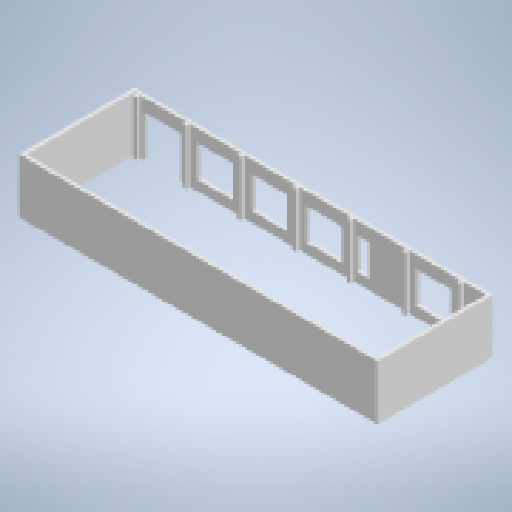
# Autodesk Inventor part: Part1
Saved by Autodesk Inventor 2024.2 (Build 282272000, 272)
## iProperties
Created: 2024-04-05
Part Number: Part1
Material: Generic
Document SubType Name: Modeling
Designer: admin
Density: 1 g/cm^3
Appearance: Default
Author: admin
Autodesk Inventor part; units mm, degrees
ref_plane "YZ Plane" through (0, 0, 0) normal (1, 0, 0) x (0, 1, 0)
ref_plane "XZ Plane" through (0, 0, 0) normal (0, 1, 0) x (-1, 0, 0)
ref_plane "XY Plane" through (0, 0, 0) normal (0, 0, 1) x (1, 0, 0)
sketch "Sketch1" plane through (0, 0, 0) normal (0, 1, 0) x (-1, 0, 0)
  line L0 (19320, -5950) -> (-19320, -5950)
  line L1 (-19320, -5950) -> (-19320, 5950)
  line L2 (-19320, 5950) -> (19320, 5950)
  line L3 (19320, 5950) -> (19320, -5950)
  line L4 (19320, -5950) -> (-19320, 5950) construction
  line L5 (-19320, -5950) -> (19320, 5950) construction
  line L6 (-19720, -6350) -> (19720, -6350)
  line L7 (19720, -6350) -> (19720, 6350)
  line L8 (19720, 6350) -> (-19720, 6350)
  line L9 (-19720, 6350) -> (-19720, -6350)
  line L10 (-16470, -5950) -> (-16870, -5950)
  line L11 (-16870, -5950) -> (-16870, -5550)
  line L12 (-16870, -5550) -> (-16470, -5550)
  line L13 (-16470, -5550) -> (-16470, -5950)
  line L14 (-16470, -5950) -> (-16870, -5550) construction
  line L15 (-16870, -5950) -> (-16470, -5550) construction
  line L16 (-16470, 5850) -> (-16870, 5850)
  line L17 (-16870, 5850) -> (-16870, 5950)
  line L18 (-16870, 5950) -> (-16470, 5950)
  line L19 (-16470, 5950) -> (-16470, 5850)
  line L20 (-16470, 5850) -> (-16870, 5950) construction
  line L21 (-16870, 5850) -> (-16470, 5950) construction
  line L22 (-10499, -5950) -> (-10899, -5950)
  line L23 (-10899, -5950) -> (-10899, -5550)
  line L24 (-10899, -5550) -> (-10499, -5550)
  line L25 (-10499, -5550) -> (-10499, -5950)
  line L26 (-10499, -5950) -> (-10899, -5550) construction
  line L27 (-10899, -5950) -> (-10499, -5550) construction
  line L28 (-4427, -5950) -> (-4827, -5950)
  line L29 (-4827, -5950) -> (-4827, -5550)
  line L30 (-4827, -5550) -> (-4427, -5550)
  line L31 (-4427, -5550) -> (-4427, -5950)
  line L32 (-4427, -5950) -> (-4827, -5550) construction
  line L33 (-4827, -5950) -> (-4427, -5550) construction
  line L34 (1573, -5950) -> (1173, -5950)
  line L35 (1173, -5950) -> (1173, -5550)
  line L36 (1173, -5550) -> (1573, -5550)
  line L37 (1573, -5550) -> (1573, -5950)
  line L38 (1573, -5950) -> (1173, -5550) construction
  line L39 (1173, -5950) -> (1573, -5550) construction
  line L40 (7598, -5950) -> (7198, -5950)
  line L41 (7198, -5950) -> (7198, -5550)
  line L42 (7198, -5550) -> (7598, -5550)
  line L43 (7598, -5550) -> (7598, -5950)
  line L44 (7598, -5950) -> (7198, -5550) construction
  line L45 (7198, -5950) -> (7598, -5550) construction
  line L46 (13628, -5950) -> (13228, -5950)
  line L47 (13228, -5950) -> (13228, -5550)
  line L48 (13228, -5550) -> (13628, -5550)
  line L49 (13628, -5550) -> (13628, -5950)
  line L50 (13628, -5950) -> (13228, -5550) construction
  line L51 (13228, -5950) -> (13628, -5550) construction
  line L52 (19118, -5950) -> (18718, -5950)
  line L53 (18718, -5950) -> (18718, -5550)
  line L54 (18718, -5550) -> (19118, -5550)
  line L55 (19118, -5550) -> (19118, -5950)
  line L56 (19118, -5950) -> (18718, -5550) construction
  line L57 (18718, -5950) -> (19118, -5550) construction
  line L58 (19320, -5950) -> (19720, -5950)
  line L59 (-19320, -5950) -> (-19720, -5950)
  line L60 (-19320, 5950) -> (-19720, 5950)
  line L61 (19320, 5950) -> (19720, 5950)
  point P0 (0, 0)
  point P1 (-16670, -5750)
  point P2 (-16670, 5900)
  point P3 (-16870, 5950)
  point P4 (-16470, 5950)
  point P5 (-10699, -5750)
  point P6 (-4627, -5750)
  point P7 (1373, -5750)
  point P8 (7398, -5750)
  point P9 (13428, -5750)
  point P10 (18918, -5750)
  dimension "d0" = 38640
  dimension "d1" = 11900
  dimension "d2" = 400
  dimension "d3" = 400
  dimension "d4" = 400
  dimension "d5" = 2450
  dimension "d6" = 100
  dimension "d35" = 6030
  dimension "d37" = 5490
  dimension "d38" = 6025
  dimension "d39" = 6000
  dimension "d40" = 6072
  dimension "d41" = 5971
  dimension "d42" = 202
  constraints: 124 end point, 20 parallel, 18 midpoint, 13 equal length, 13 perpendicular, 9 collinear, 9 horizontal, 5 point on line, 3 other
  measures "d0" distance of L1.end L2.end
  measures "d1" distance of L0.end L1.end
  measures "d2" distance between parallel lines of L0 L6
  measures "d3" distance of L11.end L12.end
  measures "d4" distance of L10.end L11.end
  measures "d5" distance between parallel lines of L1 L11
  measures "d6" distance of L18.end L16.start
  measures "d35" distance between parallel lines of L43 L49
  measures "d37" distance between parallel lines of L49 L55
  measures "d38" distance between parallel lines of L37 L43
  measures "d39" distance between parallel lines of L31 L37
  measures "d40" distance between parallel lines of L25 L31
  measures "d41" distance between parallel lines of L13 L25
  measures "d42" distance between parallel lines of L3 L55
extrude "Extrusion1" add sketch "Sketch1" along normal blind 6000 contours L58 L7 L6 L9 L59 L0 | L0 L53 L54 L55 | L0 L47 L48 L49 | L0 L41 L42 L43 | L11 L12 L13 L0 | L0 L35 L36 L37 | L23 L24 L25 L0 | L0 L29 L30 L31
sketch "Sketch2" plane through (19720, 0, -6350) normal (0, 0, -1) x (-1, 0, 0)
  line L0 (0, 0) -> (39440, 0) projected
  line L1 (39440, 0) -> (39440, 6000) projected
  line L2 (0, 6000) -> (39440, 6000) projected
  line L3 (0, 0) -> (0, 6000) projected
  line L4 (33938, 4600) -> (37938, 4600)
  line L5 (37938, 4600) -> (37938, 0)
  line L6 (37938, 0) -> (33938, 0)
  line L7 (33938, 0) -> (33938, 4600)
  line L8 (28218, 4600) -> (32118, 4600)
  line L9 (32118, 4600) -> (32118, 1100)
  line L10 (32118, 1100) -> (28218, 1100)
  line L11 (28218, 1100) -> (28218, 4600)
  line L12 (22193, 4600) -> (26093, 4600)
  line L13 (26093, 4600) -> (26093, 1100)
  line L14 (26093, 1100) -> (22193, 1100)
  line L15 (22193, 1100) -> (22193, 4600)
  line L16 (16193, 4600) -> (20093, 4600)
  line L17 (20093, 4600) -> (20093, 1100)
  line L18 (20093, 1100) -> (16193, 1100)
  line L19 (16193, 1100) -> (16193, 4600)
  line L20 (4171, 4600) -> (8071, 4600)
  line L21 (8071, 4600) -> (8071, 1100)
  line L22 (8071, 1100) -> (4171, 1100)
  line L23 (4171, 1100) -> (4171, 4600)
  line L24 (13263, 4600) -> (14533, 4600)
  line L25 (14533, 4600) -> (14533, 1100)
  line L26 (14533, 1100) -> (13263, 1100)
  line L27 (13263, 1100) -> (13263, 4600)
  line L28 (3250, 0) -> (3250, 6000) projected
  line L29 (8821, 0) -> (8821, 6000) projected
  line L30 (15293, 0) -> (15293, 6000) projected
  line L31 (21293, 0) -> (21293, 6000) projected
  line L32 (27318, 0) -> (27318, 6000) projected
  line L33 (38438, 0) -> (38438, 6000) projected
  line L34 (9221, 0) -> (9221, 6000) projected
  point P0 (19720, 0)
  dimension "d16" = 3900
  dimension "d17" = 1100
  dimension "d18" = 921
  dimension "d19" = 3500
  dimension "d43" = 750
  dimension "d44" = 900
  dimension "d45" = 900
  dimension "d46" = 900
  dimension "d47" = 4600
  dimension "d48" = 4000
  dimension "d49" = 500
  dimension "d50" = 1270
  dimension "d54" = 760
  constraints: 48 end point, 12 parallel, 8 point on line, 6 horizontal, 6 perpendicular, 3 collinear, 3 other
  measures "d16" distance of L20.start L20.end
  measures "d17" distance of the line from the sketch origin of L22
  measures "d18" distance between parallel lines of L23 L28
  measures "d19" distance of L22.end L20.start
  measures "d43" distance between parallel lines of L21 L29
  measures "d44" distance between parallel lines of L19 L30
  measures "d45" distance between parallel lines of L31 L15
  measures "d46" distance between parallel lines of L32 L11
  measures "d47" distance of L4.end L5.end
  measures "d48" distance of L4.start L4.end
  measures "d49" distance between parallel lines of L33 L5
  measures "d50" distance of L24.start L24.end
  measures "d54" distance between parallel lines of L30 L25
extrude "Extrusion2" cut sketch "Sketch2" against normal up to surface (400 mm away) contours L7 L4 L5 L0 | L8 L9 L10 L11 | L12 L13 L14 L15 | L16 L17 L18 L19 | L20 L21 L22 L23 | L24 L25 L26 L27
extrude "Extrusion3" add sketch "Sketch1" along normal blind 6000 separate body contours L2 L60 L9 L8 L7 L61
body "Solid1"
body "Solid2"
